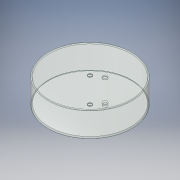
# Autodesk Inventor part: Tank
Saved by Autodesk Inventor 2017 (Build 210142000, 142)
## iProperties
Part Number: Tank
Material: Glas
Document SubType Name: Modeling
Designer: OleSi
Density: 2.18 g/cm^3
Appearance: Klar
Mass: 78.1655 g
Surface Area: 478.631 cm^2
Volume: 35.8558 cm^3
Author: OleSi
Autodesk Inventor part; units mm, degrees
ref_plane "YZ Plane" through (0, 0, 0) normal (1, 0, 0) x (0, 1, 0)
ref_plane "XZ Plane" through (0, 0, 0) normal (0, 1, 0) x (-1, 0, 0)
ref_plane "XY Plane" through (0, 0, 0) normal (0, 0, 1) x (1, 0, 0)
sketch "Skizze2" plane through (0, 0, 0) normal (0, 0, 1) x (1, 0, 0)
  circle A0 centre (0, 0) radius 50
  dimension "d2" = 100
  constraints: 1 centre point, 1 coincident
  measures "d2" diameter of A0
extrude "Extrusion1" add sketch "Skizze2" along normal blind 30
shell "Wandung1" thickness 1.5 removed faces 0
fillet "Rundung1" radius 1 1 edges at (-50, 0, 30)
chamfer "Fase1" distance 0.5 angle 45 1 edges at (-50, 0, 0)
sketch "Skizze4" plane through (0, 0, 30) normal (0, 0, 1) x (1, 0, 0)
  circle A0 centre (10, 8) radius 3.75
  point P0 (0, 0)
  point P1 (0, 0)
  dimension "d12" = 7.5
  constraints: 1 centre point
  measures "d12" diameter of A0
hole "Bohrung1" at (10, 8, 30) direction (0, 0, -1) diameter 5 end through all
sketch "Skizze5" plane through (0, 0, 30) normal (0, 0, 1) x (1, 0, 0)
  circle A0 centre (0, 0) radius 2
  circle A1 centre (0, 0) radius 2.5
  dimension "d20" = 5
  dimension "d31" = 4
  constraints: 2 centre point, 2 coincident
  measures "d20" diameter of A1
  measures "d31" diameter of A0
extrude "Extrusion3" add sketch "Skizze5" along normal blind 0.5
sketch "Skizze6" plane through (0, 0, 0) normal (0, 0, -1) x (-1, 0, 0)
  circle A0 centre (0, 0) radius 2.5 projected
  circle A1 centre (0, 0) radius 2
  circle A2 centre (0, 0) radius 2.5
  dimension "d23" = 4
  dimension "d24" = 5
  constraints: 2 centre point, 2 coincident
  measures "d23" diameter of A1
  measures "d24" diameter of A2
extrude "Extrusion4" cut sketch "Skizze6" against normal blind 0.5
sketch "Skizze7" plane through (0, 0, 28.5) normal (0, 0, -1) x (-1, 0, 0)
  circle A0 centre (-10, 8) radius 3.75
  circle A1 centre (-10, 8) radius 2.5
  circle A2 centre (-10, 8) radius 2.75
  point P0 (0, 0)
  dimension "d27" = 5.5
  dimension "d30" = 5
  constraints: 3 centre point, 2 coincident
  measures "d27" diameter of A2
  measures "d30" diameter of A1
extrude "Extrusion5" add sketch "Skizze7" along normal blind 25 contours A1 | A2
